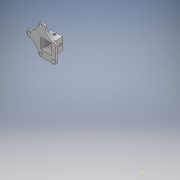
# Autodesk Inventor part: overview
Saved by Autodesk Inventor 2018 (Build 220112000, 112)
## iProperties
Created: 2018-10-10
Part Number: overview
Material: Generic
Document SubType Name: Modeling
Designer: Iek Man Lei
Density: 1 g/cm^3
Appearance: Default
Author: Iek Man Lei
Autodesk Inventor part; units mm, degrees
ref_plane "YZ Plane" through (0, 0, 0) normal (1, 0, 0) x (0, 1, 0)
ref_plane "XZ Plane" through (0, 0, 0) normal (0, 1, 0) x (-1, 0, 0)
ref_plane "XY Plane" through (0, 0, 0) normal (0, 0, 1) x (1, 0, 0)
sketch "Sketch1" plane through (0, 0, 0) normal (0, 1, 0) x (-1, 0, 0)
  line L0 (245.5, 243.75) -> (-204.5, 243.75)
  line L1 (-204.5, 243.75) -> (-204.5, -206.25)
  line L2 (-204.5, -206.25) -> (245.5, -206.25)
  line L3 (245.5, -206.25) -> (245.5, 243.75)
  circle A0 centre (233, 231.25) radius 3.3
  circle A1 centre (233, 206.25) radius 3.3
  circle A2 centre (233, 181.25) radius 3.3
  circle A3 centre (233, 156.25) radius 3.3
  circle A4 centre (233, 131.25) radius 3.3
  circle A5 centre (233, 106.25) radius 3.3
  circle A6 centre (233, 81.25) radius 3.3
  circle A7 centre (233, 56.25) radius 3.3
  circle A8 centre (233, 31.25) radius 3.3
  circle A9 centre (233, 6.25) radius 3.3
  circle A10 centre (233, -18.75) radius 3.3
  circle A11 centre (233, -43.75) radius 3.3
  circle A12 centre (233, -68.75) radius 3.3
  circle A13 centre (233, -93.75) radius 3.3
  circle A14 centre (233, -118.75) radius 3.3
  circle A15 centre (233, -143.75) radius 3.3
  circle A16 centre (233, -168.75) radius 3.3
  circle A17 centre (233, -193.75) radius 3.3
  circle A18 centre (208, 231.25) radius 3.3
  circle A19 centre (208, 206.25) radius 3.3
  circle A20 centre (208, 181.25) radius 3.3
  circle A21 centre (208, 156.25) radius 3.3
  circle A22 centre (208, 131.25) radius 3.3
  circle A23 centre (208, 106.25) radius 3.3
  circle A24 centre (208, 81.25) radius 3.3
  circle A25 centre (208, 56.25) radius 3.3
  circle A26 centre (208, 31.25) radius 3.3
  circle A27 centre (208, 6.25) radius 3.3
  circle A28 centre (208, -18.75) radius 3.3
  circle A29 centre (208, -43.75) radius 3.3
  circle A30 centre (208, -68.75) radius 3.3
  circle A31 centre (208, -93.75) radius 3.3
  circle A32 centre (208, -118.75) radius 3.3
  circle A33 centre (208, -143.75) radius 3.3
  circle A34 centre (208, -168.75) radius 3.3
  circle A35 centre (208, -193.75) radius 3.3
  circle A36 centre (183, 231.25) radius 3.3
  circle A37 centre (183, 206.25) radius 3.3
  circle A38 centre (183, 181.25) radius 3.3
  circle A39 centre (183, 156.25) radius 3.3
  circle A40 centre (183, 131.25) radius 3.3
  circle A41 centre (183, 106.25) radius 3.3
  circle A42 centre (183, 81.25) radius 3.3
  circle A43 centre (183, 56.25) radius 3.3
  circle A44 centre (183, 31.25) radius 3.3
  circle A45 centre (183, 6.25) radius 3.3
  circle A46 centre (183, -18.75) radius 3.3
  circle A47 centre (183, -43.75) radius 3.3
  circle A48 centre (183, -68.75) radius 3.3
  circle A49 centre (183, -93.75) radius 3.3
  circle A50 centre (183, -118.75) radius 3.3
  circle A51 centre (183, -143.75) radius 3.3
  circle A52 centre (183, -168.75) radius 3.3
  circle A53 centre (183, -193.75) radius 3.3
  circle A54 centre (158, 231.25) radius 3.3
  circle A55 centre (158, 206.25) radius 3.3
  circle A56 centre (158, 181.25) radius 3.3
  circle A57 centre (158, 156.25) radius 3.3
  circle A58 centre (158, 131.25) radius 3.3
  circle A59 centre (158, 106.25) radius 3.3
  circle A60 centre (158, 81.25) radius 3.3
  circle A61 centre (158, 56.25) radius 3.3
  circle A62 centre (158, 31.25) radius 3.3
  circle A63 centre (158, 6.25) radius 3.3
  circle A64 centre (158, -18.75) radius 3.3
  circle A65 centre (158, -43.75) radius 3.3
  circle A66 centre (158, -68.75) radius 3.3
  circle A67 centre (158, -93.75) radius 3.3
  circle A68 centre (158, -118.75) radius 3.3
  circle A69 centre (158, -143.75) radius 3.3
  circle A70 centre (158, -168.75) radius 3.3
  circle A71 centre (158, -193.75) radius 3.3
  circle A72 centre (133, 231.25) radius 3.3
  circle A73 centre (133, 206.25) radius 3.3
  circle A74 centre (133, 181.25) radius 3.3
  circle A75 centre (133, 156.25) radius 3.3
  circle A76 centre (133, 131.25) radius 3.3
  circle A77 centre (133, 106.25) radius 3.3
  circle A78 centre (133, 81.25) radius 3.3
  circle A79 centre (133, 56.25) radius 3.3
  circle A80 centre (133, 31.25) radius 3.3
  circle A81 centre (133, 6.25) radius 3.3
  circle A82 centre (133, -18.75) radius 3.3
  circle A83 centre (133, -43.75) radius 3.3
  circle A84 centre (133, -68.75) radius 3.3
  circle A85 centre (133, -93.75) radius 3.3
  circle A86 centre (133, -118.75) radius 3.3
  circle A87 centre (133, -143.75) radius 3.3
  circle A88 centre (133, -168.75) radius 3.3
  circle A89 centre (133, -193.75) radius 3.3
  circle A90 centre (108, 231.25) radius 3.3
  circle A91 centre (108, 206.25) radius 3.3
  circle A92 centre (108, 181.25) radius 3.3
  circle A93 centre (108, 156.25) radius 3.3
  circle A94 centre (108, 131.25) radius 3.3
  circle A95 centre (108, 106.25) radius 3.3
  circle A96 centre (108, 81.25) radius 3.3
  circle A97 centre (108, 56.25) radius 3.3
  circle A98 centre (108, 31.25) radius 3.3
  circle A99 centre (108, 6.25) radius 3.3
  circle A100 centre (108, -18.75) radius 3.3
  circle A101 centre (108, -43.75) radius 3.3
  circle A102 centre (108, -68.75) radius 3.3
  circle A103 centre (108, -93.75) radius 3.3
  circle A104 centre (108, -118.75) radius 3.3
  circle A105 centre (108, -143.75) radius 3.3
  circle A106 centre (108, -168.75) radius 3.3
  circle A107 centre (108, -193.75) radius 3.3
  circle A108 centre (83, 231.25) radius 3.3
  circle A109 centre (83, 206.25) radius 3.3
  circle A110 centre (83, 181.25) radius 3.3
  circle A111 centre (83, 156.25) radius 3.3
  circle A112 centre (83, 131.25) radius 3.3
  circle A113 centre (83, 106.25) radius 3.3
  circle A114 centre (83, 81.25) radius 3.3
  circle A115 centre (83, 56.25) radius 3.3
  circle A116 centre (83, 31.25) radius 3.3
  circle A117 centre (83, 6.25) radius 3.3
  circle A118 centre (83, -18.75) radius 3.3
  circle A119 centre (83, -43.75) radius 3.3
  circle A120 centre (83, -68.75) radius 3.3
  circle A121 centre (83, -93.75) radius 3.3
  circle A122 centre (83, -118.75) radius 3.3
  circle A123 centre (83, -143.75) radius 3.3
  circle A124 centre (83, -168.75) radius 3.3
  circle A125 centre (83, -193.75) radius 3.3
  circle A126 centre (58, 231.25) radius 3.3
  circle A127 centre (58, 206.25) radius 3.3
  circle A128 centre (58, 181.25) radius 3.3
  circle A129 centre (58, 156.25) radius 3.3
  circle A130 centre (58, 131.25) radius 3.3
  circle A131 centre (58, 106.25) radius 3.3
  circle A132 centre (58, 81.25) radius 3.3
  circle A133 centre (58, 56.25) radius 3.3
  circle A134 centre (58, 31.25) radius 3.3
  circle A135 centre (58, 6.25) radius 3.3
  circle A136 centre (58, -18.75) radius 3.3
  circle A137 centre (58, -43.75) radius 3.3
  circle A138 centre (58, -68.75) radius 3.3
  circle A139 centre (58, -93.75) radius 3.3
  circle A140 centre (58, -118.75) radius 3.3
  circle A141 centre (58, -143.75) radius 3.3
  circle A142 centre (58, -168.75) radius 3.3
  circle A143 centre (58, -193.75) radius 3.3
  circle A144 centre (33, 231.25) radius 3.3
  circle A145 centre (33, 206.25) radius 3.3
  circle A146 centre (33, 181.25) radius 3.3
  circle A147 centre (33, 156.25) radius 3.3
  circle A148 centre (33, 131.25) radius 3.3
  circle A149 centre (33, 106.25) radius 3.3
  circle A150 centre (33, 81.25) radius 3.3
  circle A151 centre (33, 56.25) radius 3.3
  circle A152 centre (33, 31.25) radius 3.3
  circle A153 centre (33, 6.25) radius 3.3
  circle A154 centre (33, -18.75) radius 3.3
  circle A155 centre (33, -43.75) radius 3.3
  circle A156 centre (33, -68.75) radius 3.3
  circle A157 centre (33, -93.75) radius 3.3
  circle A158 centre (33, -118.75) radius 3.3
  circle A159 centre (33, -143.75) radius 3.3
  circle A160 centre (33, -168.75) radius 3.3
  circle A161 centre (33, -193.75) radius 3.3
  circle A162 centre (8, 231.25) radius 3.3
  circle A163 centre (8, 206.25) radius 3.3
  circle A164 centre (8, 181.25) radius 3.3
  circle A165 centre (8, 156.25) radius 3.3
  circle A166 centre (8, 131.25) radius 3.3
  circle A167 centre (8, 106.25) radius 3.3
  circle A168 centre (8, 81.25) radius 3.3
  circle A169 centre (8, 56.25) radius 3.3
  circle A170 centre (8, 31.25) radius 3.3
  circle A171 centre (8, 6.25) radius 3.3
  circle A172 centre (8, -18.75) radius 3.3
  circle A173 centre (8, -43.75) radius 3.3
  circle A174 centre (8, -68.75) radius 3.3
  circle A175 centre (8, -93.75) radius 3.3
  circle A176 centre (8, -118.75) radius 3.3
  circle A177 centre (8, -143.75) radius 3.3
  circle A178 centre (8, -168.75) radius 3.3
  circle A179 centre (8, -193.75) radius 3.3
  circle A180 centre (-17, 231.25) radius 3.3
  circle A181 centre (-17, 206.25) radius 3.3
  circle A182 centre (-17, 181.25) radius 3.3
  circle A183 centre (-17, 156.25) radius 3.3
  circle A184 centre (-17, 131.25) radius 3.3
  circle A185 centre (-17, 106.25) radius 3.3
  circle A186 centre (-17, 81.25) radius 3.3
  circle A187 centre (-17, 56.25) radius 3.3
  circle A188 centre (-17, 31.25) radius 3.3
  circle A189 centre (-17, 6.25) radius 3.3
  circle A190 centre (-17, -18.75) radius 3.3
  circle A191 centre (-17, -43.75) radius 3.3
  circle A192 centre (-17, -68.75) radius 3.3
  circle A193 centre (-17, -93.75) radius 3.3
  circle A194 centre (-17, -118.75) radius 3.3
  circle A195 centre (-17, -143.75) radius 3.3
  circle A196 centre (-17, -168.75) radius 3.3
  circle A197 centre (-17, -193.75) radius 3.3
  circle A198 centre (-42, 231.25) radius 3.3
  circle A199 centre (-42, 206.25) radius 3.3
  circle A200 centre (-42, 181.25) radius 3.3
  circle A201 centre (-42, 156.25) radius 3.3
  circle A202 centre (-42, 131.25) radius 3.3
  circle A203 centre (-42, 106.25) radius 3.3
  circle A204 centre (-42, 81.25) radius 3.3
  circle A205 centre (-42, 56.25) radius 3.3
  circle A206 centre (-42, 31.25) radius 3.3
  circle A207 centre (-42, 6.25) radius 3.3
  circle A208 centre (-42, -18.75) radius 3.3
  circle A209 centre (-42, -43.75) radius 3.3
  circle A210 centre (-42, -68.75) radius 3.3
  circle A211 centre (-42, -93.75) radius 3.3
  circle A212 centre (-42, -118.75) radius 3.3
  circle A213 centre (-42, -143.75) radius 3.3
  circle A214 centre (-42, -168.75) radius 3.3
  circle A215 centre (-42, -193.75) radius 3.3
  circle A216 centre (-67, 231.25) radius 3.3
  circle A217 centre (-67, 206.25) radius 3.3
  circle A218 centre (-67, 181.25) radius 3.3
  circle A219 centre (-67, 156.25) radius 3.3
  circle A220 centre (-67, 131.25) radius 3.3
  circle A221 centre (-67, 106.25) radius 3.3
  circle A222 centre (-67, 81.25) radius 3.3
  circle A223 centre (-67, 56.25) radius 3.3
  circle A224 centre (-67, 31.25) radius 3.3
  circle A225 centre (-67, 6.25) radius 3.3
  circle A226 centre (-67, -18.75) radius 3.3
  circle A227 centre (-67, -43.75) radius 3.3
  circle A228 centre (-67, -68.75) radius 3.3
  circle A229 centre (-67, -93.75) radius 3.3
  circle A230 centre (-67, -118.75) radius 3.3
  circle A231 centre (-67, -143.75) radius 3.3
  circle A232 centre (-67, -168.75) radius 3.3
  circle A233 centre (-67, -193.75) radius 3.3
  circle A234 centre (-92, 231.25) radius 3.3
  circle A235 centre (-92, 206.25) radius 3.3
  circle A236 centre (-92, 181.25) radius 3.3
  circle A237 centre (-92, 156.25) radius 3.3
  circle A238 centre (-92, 131.25) radius 3.3
  circle A239 centre (-92, 106.25) radius 3.3
  circle A240 centre (-92, 81.25) radius 3.3
  circle A241 centre (-92, 56.25) radius 3.3
  circle A242 centre (-92, 31.25) radius 3.3
  circle A243 centre (-92, 6.25) radius 3.3
  circle A244 centre (-92, -18.75) radius 3.3
  circle A245 centre (-92, -43.75) radius 3.3
  circle A246 centre (-92, -68.75) radius 3.3
  circle A247 centre (-92, -93.75) radius 3.3
  circle A248 centre (-92, -118.75) radius 3.3
  circle A249 centre (-92, -143.75) radius 3.3
  circle A250 centre (-92, -168.75) radius 3.3
  circle A251 centre (-92, -193.75) radius 3.3
  circle A252 centre (-117, 231.25) radius 3.3
  circle A253 centre (-117, 206.25) radius 3.3
  circle A254 centre (-117, 181.25) radius 3.3
  circle A255 centre (-117, 156.25) radius 3.3
  circle A256 centre (-117, 131.25) radius 3.3
  circle A257 centre (-117, 106.25) radius 3.3
  circle A258 centre (-117, 81.25) radius 3.3
  circle A259 centre (-117, 56.25) radius 3.3
  circle A260 centre (-117, 31.25) radius 3.3
  circle A261 centre (-117, 6.25) radius 3.3
  circle A262 centre (-117, -18.75) radius 3.3
  circle A263 centre (-117, -43.75) radius 3.3
  circle A264 centre (-117, -68.75) radius 3.3
  circle A265 centre (-117, -93.75) radius 3.3
  circle A266 centre (-117, -118.75) radius 3.3
  circle A267 centre (-117, -143.75) radius 3.3
  circle A268 centre (-117, -168.75) radius 3.3
  circle A269 centre (-117, -193.75) radius 3.3
  circle A270 centre (-142, 231.25) radius 3.3
  circle A271 centre (-142, 206.25) radius 3.3
  circle A272 centre (-142, 181.25) radius 3.3
  circle A273 centre (-142, 156.25) radius 3.3
  circle A274 centre (-142, 131.25) radius 3.3
  circle A275 centre (-142, 106.25) radius 3.3
  circle A276 centre (-142, 81.25) radius 3.3
  circle A277 centre (-142, 56.25) radius 3.3
  circle A278 centre (-142, 31.25) radius 3.3
  circle A279 centre (-142, 6.25) radius 3.3
  circle A280 centre (-142, -18.75) radius 3.3
  circle A281 centre (-142, -43.75) radius 3.3
  circle A282 centre (-142, -68.75) radius 3.3
  circle A283 centre (-142, -93.75) radius 3.3
  circle A284 centre (-142, -118.75) radius 3.3
  circle A285 centre (-142, -143.75) radius 3.3
  circle A286 centre (-142, -168.75) radius 3.3
  circle A287 centre (-142, -193.75) radius 3.3
  circle A288 centre (-167, 231.25) radius 3.3
  circle A289 centre (-167, 206.25) radius 3.3
  circle A290 centre (-167, 181.25) radius 3.3
  circle A291 centre (-167, 156.25) radius 3.3
  circle A292 centre (-167, 131.25) radius 3.3
  circle A293 centre (-167, 106.25) radius 3.3
  circle A294 centre (-167, 81.25) radius 3.3
  circle A295 centre (-167, 56.25) radius 3.3
  circle A296 centre (-167, 31.25) radius 3.3
  circle A297 centre (-167, 6.25) radius 3.3
  circle A298 centre (-167, -18.75) radius 3.3
  circle A299 centre (-167, -43.75) radius 3.3
  circle A300 centre (-167, -68.75) radius 3.3
  circle A301 centre (-167, -93.75) radius 3.3
  circle A302 centre (-167, -118.75) radius 3.3
  circle A303 centre (-167, -143.75) radius 3.3
  circle A304 centre (-167, -168.75) radius 3.3
  circle A305 centre (-167, -193.75) radius 3.3
  circle A306 centre (-192, 231.25) radius 3.3
  circle A307 centre (-192, 206.25) radius 3.3
  circle A308 centre (-192, 181.25) radius 3.3
  circle A309 centre (-192, 156.25) radius 3.3
  circle A310 centre (-192, 131.25) radius 3.3
  circle A311 centre (-192, 106.25) radius 3.3
  circle A312 centre (-192, 81.25) radius 3.3
  circle A313 centre (-192, 56.25) radius 3.3
  circle A314 centre (-192, 31.25) radius 3.3
  circle A315 centre (-192, 6.25) radius 3.3
  circle A316 centre (-192, -18.75) radius 3.3
  circle A317 centre (-192, -43.75) radius 3.3
  circle A318 centre (-192, -68.75) radius 3.3
  circle A319 centre (-192, -93.75) radius 3.3
  circle A320 centre (-192, -118.75) radius 3.3
  circle A321 centre (-192, -143.75) radius 3.3
  circle A322 centre (-192, -168.75) radius 3.3
  circle A323 centre (-192, -193.75) radius 3.3
  line L4 (208, 241.25) -> (168, 241.25)
  line L5 (168, 241.25) -> (168, 221.25)
  line L6 (168, 221.25) -> (208, 221.25)
  line L7 (208, 221.25) -> (208, 241.25)
  line L8 (208, -203.75) -> (168, -203.75)
  line L9 (168, -203.75) -> (168, -183.75)
  line L10 (168, -183.75) -> (208, -183.75)
  line L11 (208, -183.75) -> (208, -203.75)
  line L12 (188, 221.25) -> (168, 221.25)
  line L13 (168, 221.25) -> (168, -183.75)
  line L14 (168, -183.75) -> (188, -183.75)
  line L15 (188, -183.75) -> (188, 221.25)
  line L16 (168, -5.25) -> (188, -5.25)
  line L17 (188, -5.25) -> (188, 42.75)
  line L18 (188, 42.75) -> (168, 42.75)
  line L19 (168, 42.75) -> (168, -5.25)
  line L20 (168, 42.75) -> (188, 42.75)
  line L21 (188, 42.75) -> (188, 65.75)
  line L22 (188, 65.75) -> (168, 65.75)
  line L23 (168, 65.75) -> (168, 42.75)
  line L24 (188, -5.25) -> (168, -5.25)
  line L25 (168, -5.25) -> (168, -28.25)
  line L26 (168, -28.25) -> (188, -28.25)
  line L27 (188, -28.25) -> (188, -5.25)
  line L28 (188, 65.75) -> (168, 65.75)
  line L29 (168, 65.75) -> (168, 113.75)
  line L30 (168, 113.75) -> (188, 113.75)
  line L31 (188, 113.75) -> (188, 65.75)
  line L32 (188, 113.75) -> (168, 113.75)
  line L33 (168, 113.75) -> (168, 136.75)
  line L34 (168, 136.75) -> (188, 136.75)
  line L35 (188, 136.75) -> (188, 113.75)
  line L36 (188, 135.25) -> (208, 135.25)
  line L37 (208, 135.25) -> (208, 115.25)
  line L38 (208, 115.25) -> (188, 115.25)
  line L39 (188, 115.25) -> (188, 135.25)
  line L40 (177.7, 100.95) -> (238.3, 100.95)
  line L41 (238.3, 100.95) -> (238.3, 161.55)
  line L42 (238.3, 161.55) -> (177.7, 161.55)
  line L43 (177.7, 161.55) -> (177.7, 100.95)
  point P0 (0, 0)
  dimension "d0" = 450
  dimension "d1" = 450
  dimension "d2" = 6.6
  dimension "d3" = 12.5
  dimension "d4" = 12.5
  dimension "d7" = 25
  dimension "d10" = 25
  dimension "d13" = 40
  dimension "d14" = 20
  dimension "d15" = 2.5
  dimension "d16" = 2.5
  dimension "d17" = 20
  dimension "d21" = 48
  dimension "d22" = 178.5
  dimension "d23" = 178.5
  dimension "d24" = 23
  dimension "d25" = 23
  dimension "d26" = 48
  dimension "d27" = 23
  dimension "d28" = 20
  dimension "d29" = 20
  dimension "d30" = 1.5
  dimension "d31" = 60.6
  dimension "d32" = 5.3
  dimension "d33" = 5.3
  dimension "d34" = 5.3
  dimension "d75" = 0
  dimension "d76" = 0
  dimension "d77" = 40
  constraints: 324 centre point, 88 end point, 22 parallel, 12 horizontal, 11 perpendicular, 8 point on line, 2 midpoint, 1 vertical, 646 other
  measures "d0" distance of L2.end L0.start
  measures "d1" distance of L1.end L2.end
  measures "d2" diameter of A0
  measures "d3" distance from line of A0.centre L3
  measures "d4" distance from line of L0 A0.centre
  measures "d7" distance of A0.centre A1.centre
  measures "d10" distance of A0.centre A18.centre
  measures "d13" distance of L6.end L5.end
  measures "d14" distance of L4.end L5.end
  measures "d15" distance between parallel lines of L0 L4
  measures "d16" distance between parallel lines of L8 L2
  measures "d17" distance of L14.end L13.end
  measures "d21" distance of L16.end L17.end
  measures "d22" distance between parallel lines of L14 L16
  measures "d23" distance between parallel lines of L12 L18
  measures "d24" distance of L21.end L17.end
  measures "d25" distance of L16.end L26.end
  measures "d26" distance of L30.end L21.end
  measures "d27" distance of L33.end L29.end
  measures "d28" distance of L37.end L38.end
  measures "d29" distance of L36.end L37.end
  measures "d30" distance between parallel lines of L38 L32
  measures "d31" distance of L40.end L41.end
  measures "d32" distance from line of L42 A3.centre
  measures "d33" distance from line of L41 A4.centre
  measures "d34" distance from line of L43 A40.centre
  measures "d75" distance between parallel lines of L5 L13
  measures "d76" distance between parallel lines of L13 L9
  measures "d77" distance of L8.start L8.end
sketch "Sketch2" plane through (0, 0, 0) normal (0, 1, 0) x (-1, 0, 0)
  point P0 (0, 0)
extrude "Extrusion1" add sketch "Sketch1" along normal blind 3 contours L42 L41 L40 L15 L38 L37 A22 L36 | L15 L34 L43 L42 | L15 L30 L43 L34 | L30 L15 L40 L43 | A22 L37 picked at (209.1, 131.25)
sketch "Sketch4" plane through (0, 3, 0) normal (0, 1, 0) x (1, 0, 0)
  line L0 (-210.25, -137.5) -> (-185.75, -137.5)
  line L1 (-185.75, -137.5) -> (-185.75, -113)
  line L2 (-185.75, -113) -> (-210.25, -113)
  line L3 (-210.25, -113) -> (-210.25, -137.5)
  line L4 (-187.75, -135.5) -> (-208.25, -135.5) projected
  line L5 (-208.25, -135.5) -> (-208.25, -115) projected
  point P0 (0, 0)
  dimension "d43" = 24.5
  dimension "d44" = 24.5
  dimension "d45" = 2
  dimension "d46" = 2
  constraints: 8 end point, 2 parallel, 1 horizontal, 1 perpendicular
  measures "d43" distance of L2.end L1.end
  measures "d44" distance of L0.end L1.end
  measures "d45" distance between parallel lines of L0 L4
  measures "d46" distance between parallel lines of L5 L3
extrude "Extrusion3" add sketch "Sketch4" along normal blind 20
sketch "Sketch5" plane through (0, 23, 0) normal (0, 1, 0) x (1, 0, 0)
  line L0 (-208.25, -135.5) -> (-187.75, -135.5)
  line L1 (-187.75, -135.5) -> (-187.75, -115)
  line L2 (-187.75, -115) -> (-208.25, -115)
  line L3 (-208.25, -115) -> (-208.25, -135.5)
  line L4 (-210.25, -113) -> (-210.25, -137.5) projected
  line L5 (-210.25, -137.5) -> (-185.75, -137.5) projected
  point P0 (0, 0)
  dimension "d49" = 20.5
  dimension "d50" = 20.5
  dimension "d51" = 2
  dimension "d52" = 2
  constraints: 8 end point, 2 parallel, 1 horizontal, 1 perpendicular
  measures "d49" distance of L2.end L1.end
  measures "d50" distance of L0.end L1.end
  measures "d51" distance between parallel lines of L4 L3
  measures "d52" distance between parallel lines of L5 L0
extrude "Extrusion4" cut sketch "Sketch5" against normal blind 25
fillet "Fillet1" [suppressed]
sketch "Sketch7" plane through (-207.25, 6, 137.5) normal (0, 0, 1) x (1, 0, 0)
  circle A0 centre (9.25, 11) radius 2.75
  line L0 (-3, 17) -> (21.5, 17) projected
  line L1 (-3, 17) -> (-3, 0) projected
  point P0 (207.25, -6)
  point P1 (0, 17)
  point P2 (18.5, 17)
  dimension "d63" = 5.5
  dimension "d64" = 6
  dimension "d65" = 12.25
  constraints: 1 centre point
  measures "d63" diameter of A0
  measures "d64" distance from line of L0 A0.centre
  measures "d65" distance from line of A0.centre L1
extrude "Extrusion6" cut sketch "Sketch7" against normal blind 25
sketch "Sketch8" plane through (-210.25, 6, 116) normal (-1, 0, 0) x (0, 0, 1)
  circle A0 centre (9.25, 11) radius 2.75
  line L0 (-3, 17) -> (21.5, 17) projected
  line L1 (-3, 17) -> (-3, 0) projected
  point P0 (-116, -6)
  point P1 (0, 17)
  point P2 (18.5, 17)
  dimension "d68" = 5.5
  dimension "d69" = 6
  dimension "d70" = 12.25
  constraints: 1 centre point
  measures "d68" diameter of A0
  measures "d69" distance from line of L0 A0.centre
  measures "d70" distance from line of A0.centre L1
extrude "Extrusion7" cut sketch "Sketch8" against normal blind 25
fillet "Fillet3" radius 1 8 edges at (-210.25, 23, 125.25) (-198, 23, 137.5) (-185.75, 23, 125.25) (-198, 23, 113) (-198, 23, 115) (-208.25, 23, 125.25) (-187.75, 23, 125.25) (-198, 23, 135.5)
fillet "Fillet4" radius 1 4 edges at (-198, 0, 135.5) (-208.25, 0, 125.25) (-187.75, 0, 125.25) (-198, 0, 115)
sketch "Sketch9" plane through (0, 3, 0) normal (0, 1, 0) x (1, 0, 0)
  line L0 (-238.3, -161.55) -> (-177.7, -161.55) projected
  circle A0 centre (-238.3, -161.55) radius 25
  line L1 (-177.7, -100.95) -> (-238.3, -100.95) projected
  circle A1 centre (-238.3, -100.95) radius 25
  point P0 (0, 0)
  dimension "d78" = 50
  dimension "d79" = 50
  constraints: 2 centre point
  measures "d78" diameter of A0
  measures "d79" diameter of A1
extrude "Extrusion8" cut sketch "Sketch9" against normal blind 25
sketch "Sketch10" plane through (0, 3, 0) normal (0, 1, 0) x (1, 0, 0)
  line L0 (-178, -125) -> (-187, -125)
  line L1 (-187, -125) -> (-187, -137.5)
  line L2 (-187, -137.5) -> (-178, -137.5)
  line L3 (-178, -137.5) -> (-178, -125)
  point P0 (0, 0)
  constraints: 8 end point, 2 parallel, 1 horizontal, 1 perpendicular
extrude "Extrusion9" add sketch "Sketch10" against normal blind 3
sketch "Sketch11" plane through (0, 3, 0) normal (0, 1, 0) x (1, 0, 0)
  line L0 (-213.3, -161.55) -> (-177.7, -161.55) projected
  circle A0 centre (-177.7, -161.55) radius 22.5
  point P0 (0, 0)
  dimension "d84" = 45
  constraints: 1 centre point
  measures "d84" diameter of A0
extrude "Extrusion10" cut sketch "Sketch11" against normal blind 3
fillet "Fillet5" radius 3 4 edges at (-210.25, 3, 125.25) (-198, 3, 113) (-185.75, 3, 125.25) (-198, 3, 137.5)
fillet "Fillet6" radius 5 7 edges at (-238.3, 1.5, 136.55) (-238.3, 1.5, 125.95) (-213.3, 1.5, 100.95) (-213.3, 1.5, 161.55) (-200.2, 1.5, 161.55) (-177.7, 1.5, 139.05) (-177.7, 1.5, 100.95)
body "Solid1"
